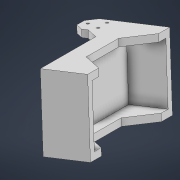
# Autodesk Inventor part: psu holder left
Saved by Autodesk Inventor 2021 (Build 250183000, 183)
## iProperties
Created: 2020-10-29
Part Number: psu holder left
Material: Generic
Document SubType Name: Modeling
Designer: brand
Density: 1 g/cm^3
Appearance: Default
Author: brand
## iProperties of the stored document _3DPrint.ipt
Created: 2020-10-29
Part Number: _3DPrint
Material: Generic
Document SubType Name: Modeling
Designer: brand
Density: 1 g/cm^3
Appearance: Default
Author: brand
Autodesk Inventor part; units mm, degrees
ref_plane "YZ Plane" through (0, 0, 0) normal (1, 0, 0) x (0, 1, 0)
ref_plane "XZ Plane" through (0, 0, 0) normal (0, 1, 0) x (-1, 0, 0)
ref_plane "XY Plane" through (0, 0, 0) normal (0, 0, 1) x (1, 0, 0)
sketch "Sketch1" plane through (0, 0, 0) normal (0, 0, 1) x (1, 0, 0)
  line L0 (0, 0) -> (0, 53.5)
  line L1 (0, 53.5) -> (30, 53.5)
  line L2 (30, 53.5) -> (30, 43.5)
  line L3 (30, 43.5) -> (10, 23.5)
  line L4 (10, 23.5) -> (10, 0)
  line L5 (-6, 0) -> (36, 0) projected
  line L6 (0, 0) -> (0, -53.5)
  line L7 (0, -53.5) -> (30, -53.5)
  line L8 (30, -53.5) -> (30, -43.5)
  line L9 (30, -43.5) -> (10, -23.5)
  line L10 (10, -23.5) -> (10, 0)
  dimension "d0" = 53.5
  dimension "d1" = 10
  dimension "d2" = 10
  dimension "d3" = 135
  dimension "d4" = 30
  constraints: 20 end point, 4 symmetric about line, 3 point on line, 2 perpendicular, 1 parallel, 1 vertical
  measures "d0" distance of L0.start L0.end
  measures "d1" distance between parallel lines of L4 L0
  measures "d2" distance of L1.end L2.end
  measures "d3" angle of L3 L2
  measures "d4" distance of L0.end L1.end
extrude "Extrusion1" add sketch "Sketch1" along normal blind 6
sketch "Sketch2" plane through (0, 0, 0) normal (0, 0, 1) x (1, 0, 0)
  line L0 (0, -53.5) -> (30, -53.5) projected
  line L1 (0, 53.5) -> (0, -53.5) projected
  line L2 (30, 53.5) -> (0, 53.5) projected
  line L3 (30, 53.5) -> (0, 53.5) projected
  line L4 (30, 53.5) -> (30, 59.5)
  line L5 (30, 59.5) -> (-6, 59.5)
  line L6 (-6, 59.5) -> (-6, -59.5)
  line L7 (-6, -59.5) -> (30, -59.5)
  line L8 (30, -59.5) -> (30, -53.5)
  point P0 (0, 0)
  dimension "d7" = 6
  dimension "d8" = 6
  dimension "d9" = 6
  constraints: 10 end point, 4 perpendicular, 1 point on line, 1 vertical
  measures "d7" distance of L7.end L0.end
  measures "d8" distance between parallel lines of L1 L6
  measures "d9" distance of L2.start L4.end
extrude "Extrusion2" add sketch "Sketch2" along normal blind 31
mirror "Mirror1" about plane through (12, 0, 31) normal (0, 0, 1) of "Extrusion1", "Extrusion2"
sketch "Sketch4" plane through (0, 0, 62) normal (0, 0, 1) x (1, 0, 0)
  line L0 (-6, 59.5) -> (-6, -59.5) construction
  line L1 (30, 59.5) -> (-6, 59.5) construction
  line L2 (-6, 59.5) -> (-31, 59.5)
  line L3 (-31, 59.5) -> (-31, 33.5)
  line L4 (-31, 33.5) -> (-6, 33.5)
  line L5 (-6, 59.5) -> (-6, -59.5) projected
  line L6 (-6, 59.5) -> (-6, 33.5)
  line L7 (-18, 22.2914) -> (-18, 69.8308) construction
  line L8 (-26.7913, 46.5) -> (-0.8939, 46.5) construction
  circle A0 centre (-18, 46.5) radius 7.5 construction
  circle A1 centre (-25.5, 46.5) radius 1.25
  circle A2 centre (-14.25, 40.0048) radius 1.25
  circle A3 centre (-14.25, 52.9952) radius 1.25
  point P0 (0, 0)
  dimension "d39" = 15
  dimension "d26" = 25
  dimension "d27" = 26
  dimension "d30" = 12
  dimension "d38" = 13
  dimension "d40" = 2.5
  dimension "d43" = 360
  constraints: 12 end point, 4 point on line, 3 centre point, 3 perpendicular, 2 horizontal, 1 horizontal alignment, 1 parallel, 9 other
  measures "d26" distance of L3.end L4.end
  measures "d27" distance of L2.end L3.end
  measures "d30" distance between parallel lines of L0 L7
  measures "d38" distance between parallel lines of L4 L8
  measures "d40" diameter of A1
extrude "Extrusion3" add sketch "Sketch4" against normal blind 6
chamfer "Chamfer1" distance 7.5 angle 45 2 edges at (-31, 33.5, 59) (-31, 59.5, 59)
chamfer "Chamfer2" distance 12.5 angle 45 1 edges at (-6, 33.5, 59)
chamfer "Chamfer3" distance 3 angle 45 2 edges at (-6, 27.25, 56) (-6, 46.5, 56)
ref_plane "Work Plane1" through (0, 0, 62) normal (-1, 0, 0) x (0, 1, 0)
equation "\"d0\" = 0.5 * width"
equation "\"d1\" = border"
equation "\"d2\" = border"
equation "\"d5\" = wall_thickness"
equation "\"d7\" = wall_thickness"
equation "\"d8\" = wall_thickness"
equation "\"d9\" = wall_thickness"
equation "\"d10\" = wall_thickness + 0.5 * depth"
equation "\"d38\" = 0.5 * d27"
equation "\"d33\" = wall_thickness"
equation "\"width\" = 107"
equation "\"border\" = 10"
equation "\"wall_thickness\" = 6"
equation "\"depth\" = 50"
body "Solid1"
